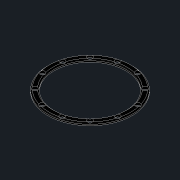
# Autodesk Inventor part: base46
Saved by Autodesk Inventor 2022 (Build 260153000, 153)
## iProperties
Created: 2021-09-01
Part Number: base46
Material: ABS プラスチック
Document SubType Name: Modeling
Designer: Yuta Kage
Density: 1.06 g/cm^3
Appearance: 滑らか - 黒
Author: Yuta Kage
Autodesk Inventor part; units mm, degrees
ref_plane "YZ Plane" through (0, 0, 0) normal (1, 0, 0) x (0, 1, 0)
ref_plane "XZ Plane" through (0, 0, 0) normal (0, 1, 0) x (-1, 0, 0)
ref_plane "XY Plane" through (0, 0, 0) normal (0, 0, 1) x (1, 0, 0)
sketch "スケッチ1" plane through (0, 0, 0) normal (0, 1, 0) x (-1, 0, 0)
  circle A0 centre (0, 0) radius 62.5 construction
  circle A1 centre (0, 0) radius 67.5
  circle A2 centre (0, 0) radius 57.5
  dimension "d0" = 125
  dimension "d1" = 5
  dimension "d2" = 5
  constraints: 3 centre point, 1 coincident
  measures "d0" diameter of A0
  measures "d1" radial gap between concentric circles of A0 A1
  measures "d2" radial gap between concentric circles of A0 A2
extrude "押し出し1" add sketch "スケッチ1" along normal blind 4
sketch "スケッチ2" plane through (0, 4, 0) normal (0, 1, 0) x (1, 0, 0)
  circle A0 centre (0, 0) radius 62.5 construction
  circle A1 centre (16.1762, -60.3704) radius 4
  circle A2 centre (44.1942, -44.1942) radius 4
  circle A3 centre (60.3704, -16.1762) radius 4
  circle A4 centre (60.3704, 16.1762) radius 4
  circle A5 centre (44.1942, 44.1942) radius 4
  circle A6 centre (16.1762, 60.3704) radius 4
  circle A7 centre (-16.1762, 60.3704) radius 4
  circle A8 centre (-44.1942, 44.1942) radius 4
  circle A9 centre (-60.3704, 16.1762) radius 4
  circle A10 centre (-60.3704, -16.1762) radius 4
  circle A11 centre (-44.1942, -44.1942) radius 4
  circle A12 centre (-16.1762, -60.3704) radius 4
  dimension "d5" = 125
  dimension "d6" = 8
  dimension "d9" = 360
  constraints: 12 centre point, 1 coincident, 1 vertical alignment, 28 other
  measures "d6" diameter of A1
extrude "押し出し2" cut sketch "スケッチ2" against normal through all
chamfer "面取り1" distance 2 angle 45 2 edges at (67.5, 4, 0) (57.5, 4, 0)
